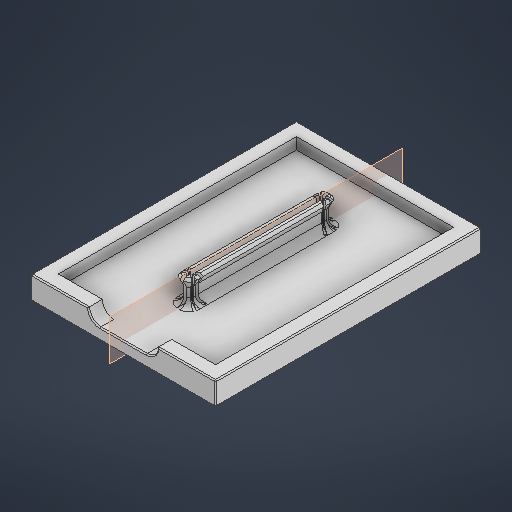
# Autodesk Inventor part: Bolt Slot Covers
Saved by Autodesk Inventor 2026.2 (Build 302298000, 298)
## iProperties
Created: 2026-05-27
Part Number: Bolt Slot Covers
Material: Generic
Document SubType Name: Modeling
Designer: mayhe
Density: 1 g/cm^3
Appearance: Default
Author: mayhe
Autodesk Inventor part; units mm, degrees
ref_plane "XZ Plane" through (0, 0, 0) normal (0, 1, 0) x (-1, 0, 0)
ref_plane "XY Plane" through (0, 0, 0) normal (0, 0, 1) x (1, 0, 0)
sketch "Sketch1" plane through (0, 0, 0) normal (0, 1, 0) x (-1, 0, 0)
  line L0 (40, 57.5) -> (-40, 57.5)
  line L1 (-40, 57.5) -> (-40, -57.5)
  line L2 (-40, -57.5) -> (40, -57.5)
  line L3 (40, -57.5) -> (40, 57.5)
  line L4 (40, 57.5) -> (-40, -57.5) construction
  line L5 (-40, 57.5) -> (40, -57.5) construction
  point P0 (0, 0)
  dimension "d0" = 80
  dimension "d1" = 115
  constraints: 12 end point, 2 midpoint, 2 parallel, 1 horizontal, 1 perpendicular
  measures "d0" distance of L2.end L1.end
  measures "d1" distance of L1.end L0.end
extrude "Extrusion1" add sketch "Sketch1" along normal mid plane 5
sketch "Sketch5" plane through (0, -2.5, 0) normal (0, -1, 0) x (1, 0, 0)
  line L0 (-43.2011, -30.2935) -> (-43.2011, 28.7129) construction
  line L1 (-43.2011, 28.7129) -> (40.8303, 28.7129) construction
  line L2 (40.8303, 28.7129) -> (40.8303, -30.2935) construction
  line L3 (40.8303, -30.2935) -> (-43.2011, -30.2935) construction
  spline S0 degree 2 poles (-3.5733, -17.3493) (-3.5733, -18.0112) (-3.8499, -18.9399) (-4.0475, -19.35) knots 0 0 0 1 2 2 2
  line L4 (-4.0475, -19.35) -> (-5.0652, -19.35)
  line L5 (-5.0652, -19.35) -> (-5.0652, -19.2907)
  spline S1 degree 2 poles (-5.0652, -19.2907) (-4.6897, -18.8905) (-4.2748, -17.8778) (-4.2748, -17.4085) knots 0 0 0 1 2 2 2
  spline S2 degree 2 poles (-4.2748, -17.4085) (-4.2748, -16.7367) (-4.833, -16.05) (-5.2924, -16.05) knots 0 0 0 1 2 2 2
  spline S3 degree 2 poles (-5.2924, -16.05) (-5.658, -16.05) (-6.1125, -16.4106) (-6.2261, -16.8009) knots 0 0 0 1 2 2 2
  spline S4 degree 2 poles (-6.2261, -16.8009) (-6.3051, -17.0825) (-6.4138, -17.5518) (-6.5027, -17.9025) knots 0 0 0 1 2 2 2
  spline S5 degree 2 poles (-6.5027, -17.9025) (-6.5867, -18.2187) (-6.8386, -18.7176) (-7.0412, -18.9103) knots 0 0 0 1 2 2 2
  spline S6 degree 2 poles (-7.0412, -18.9103) (-7.2437, -19.098) (-7.7871, -19.3055) (-8.1428, -19.3055) knots 0 0 0 1 2 2 2
  spline S7 degree 2 poles (-8.1428, -19.3055) (-8.8838, -19.3055) (-9.8866, -18.1495) (-9.8866, -17.2554) knots 0 0 0 1 2 2 2
  spline S8 degree 2 poles (-9.8866, -17.2554) (-9.8866, -16.7416) (-9.6841, -15.8327) (-9.4914, -15.4424) knots 0 0 0 1 2 2 2
  line L6 (-9.4914, -15.4424) -> (-8.5232, -15.4424)
  line L7 (-8.5232, -15.4424) -> (-8.5232, -15.5017)
  spline S9 degree 2 poles (-8.5232, -15.5017) (-8.79, -15.7931) (-9.1852, -16.7021) (-9.1852, -17.2011) knots 0 0 0 1 2 2 2
  spline S10 degree 2 poles (-9.1852, -17.2011) (-9.1852, -17.7642) (-8.6566, -18.4608) (-8.2268, -18.4608) knots 0 0 0 1 2 2 2
  spline S11 degree 2 poles (-8.2268, -18.4608) (-7.8415, -18.4608) (-7.382, -18.0507) (-7.2783, -17.6654) knots 0 0 0 1 2 2 2
  spline S12 degree 2 poles (-7.2783, -17.6654) (-7.2091, -17.4085) (-7.0313, -16.6626) (-6.9572, -16.4156) knots 0 0 0 1 2 2 2
  spline S13 degree 2 poles (-6.9572, -16.4156) (-6.7645, -15.7882) (-5.989, -15.2053) (-5.4209, -15.2053) knots 0 0 0 1 2 2 2
  spline S14 degree 2 poles (-5.4209, -15.2053) (-5.0602, -15.2053) (-4.3686, -15.4967) (-4.1266, -15.7586) knots 0 0 0 1 2 2 2
  spline S15 degree 2 poles (-4.1266, -15.7586) (-3.8598, -16.05) (-3.5733, -16.791) (-3.5733, -17.3493) knots 0 0 0 1 2 2 2
  line L8 (-3.682, -13.6541) -> (-3.682, -14.4248)
  line L9 (-3.682, -14.4248) -> (-10.0497, -14.4248)
  line L10 (-10.0497, -14.4248) -> (-10.0497, -13.6541)
  line L11 (-10.0497, -13.6541) -> (-3.682, -13.6541)
  spline S16 degree 2 poles (-5.9692, -8.7635) (-4.8132, -8.7635) (-3.5535, -9.875) (-3.5535, -10.8037) knots 0 0 0 1 2 2 2
  spline S17 degree 2 poles (-3.5535, -10.8037) (-3.5535, -11.7571) (-4.8527, -12.8489) (-5.9692, -12.8489) knots 0 0 0 1 2 2 2
  spline S18 degree 2 poles (-5.9692, -12.8489) (-7.1153, -12.8489) (-8.3849, -11.7226) (-8.3849, -10.8037) knots 0 0 0 1 2 2 2
  spline S19 degree 2 poles (-8.3849, -10.8037) (-8.3849, -9.875) (-7.1202, -8.7635) (-5.9692, -8.7635) knots 0 0 0 1 2 2 2
  spline S20 degree 2 poles (-5.9692, -9.5588) (-6.8584, -9.5588) (-7.7229, -10.206) (-7.7229, -10.8037) knots 0 0 0 1 2 2 2
  spline S21 degree 2 poles (-7.7229, -10.8037) (-7.7229, -11.4015) (-6.8584, -12.0535) (-5.9692, -12.0535) knots 0 0 0 1 2 2 2
  spline S22 degree 2 poles (-5.9692, -12.0535) (-5.1047, -12.0535) (-4.2155, -11.4015) (-4.2155, -10.8037) knots 0 0 0 1 2 2 2
  spline S23 degree 2 poles (-4.2155, -10.8037) (-4.2155, -10.2109) (-5.0899, -9.5588) (-5.9692, -9.5588) knots 0 0 0 1 2 2 2
  spline S24 degree 2 poles (-3.593, -6.5899) (-3.593, -7.2172) (-4.3093, -7.9237) (-5.0849, -7.9237) knots 0 0 0 1 2 2 2
  line L12 (-5.0849, -7.9237) -> (-7.6192, -7.9237)
  line L13 (-7.6192, -7.9237) -> (-7.6192, -8.4424)
  line L14 (-7.6192, -8.4424) -> (-8.2564, -8.4424)
  line L15 (-8.2564, -8.4424) -> (-8.2564, -7.9237)
  line L16 (-8.2564, -7.9237) -> (-9.5705, -7.9237)
  line L17 (-9.5705, -7.9237) -> (-9.5705, -7.153)
  line L18 (-9.5705, -7.153) -> (-8.2564, -7.153)
  line L19 (-8.2564, -7.153) -> (-8.2564, -5.7352)
  line L20 (-8.2564, -5.7352) -> (-7.6192, -5.7352)
  line L21 (-7.6192, -5.7352) -> (-7.6192, -7.153)
  line L22 (-7.6192, -7.153) -> (-5.4406, -7.153)
  spline S25 degree 2 poles (-5.4406, -7.153) (-5.0948, -7.153) (-4.7144, -7.1283) (-4.5514, -7.0443) knots 0 0 0 1 2 2 2
  spline S26 degree 2 poles (-4.5514, -7.0443) (-4.4081, -6.9752) (-4.2649, -6.664) (-4.2649, -6.3972) knots 0 0 0 1 2 2 2
  spline S27 degree 2 poles (-4.2649, -6.3972) (-4.2649, -6.2095) (-4.3785, -5.8587) (-4.4131, -5.7797) knots 0 0 0 1 2 2 2
  line L23 (-4.4131, -5.7797) -> (-4.4131, -5.7352)
  line L24 (-4.4131, -5.7352) -> (-3.7215, -5.7352)
  spline S28 degree 2 poles (-3.7215, -5.7352) (-3.6622, -5.9526) (-3.593, -6.3972) (-3.593, -6.5899) knots 0 0 0 1 2 2 2
  spline S29 degree 2 poles (-3.5733, -0.1085) (-3.5733, -0.7013) (-3.9734, -1.7042) (-4.3736, -2.0697) knots 0 0 0 1 2 2 2
  spline S30 degree 2 poles (-4.3736, -2.0697) (-4.7688, -2.4353) (-5.9544, -2.8354) (-6.725, -2.8354) knots 0 0 0 1 2 2 2
  spline S31 degree 2 poles (-6.725, -2.8354) (-7.4907, -2.8354) (-8.6269, -2.4452) (-9.0468, -2.0747) knots 0 0 0 1 2 2 2
  spline S32 degree 2 poles (-9.0468, -2.0747) (-9.4569, -1.7091) (-9.8866, -0.7112) (-9.8866, -0.0937) knots 0 0 0 1 2 2 2
  spline S33 degree 2 poles (-9.8866, -0.0937) (-9.8866, 0.2126) (-9.7977, 0.751) (-9.7286, 0.9783) knots 0 0 0 1 2 2 2
  spline S34 degree 2 poles (-9.7286, 0.9783) (-9.6643, 1.1759) (-9.4816, 1.5859) (-9.3729, 1.7884) knots 0 0 0 1 2 2 2
  line L25 (-9.3729, 1.7884) -> (-8.3948, 1.7884)
  line L26 (-8.3948, 1.7884) -> (-8.3948, 1.7242)
  spline S35 degree 2 poles (-8.3948, 1.7242) (-8.4936, 1.6155) (-8.7702, 1.2796) (-8.9036, 1.0375) knots 0 0 0 1 2 2 2
  spline S36 degree 2 poles (-8.9036, 1.0375) (-9.032, 0.8054) (-9.195, 0.257) (-9.195, -0.0987) knots 0 0 0 1 2 2 2
  spline S37 degree 2 poles (-9.195, -0.0987) (-9.195, -0.4889) (-8.8739, -1.1855) (-8.5677, -1.4473) knots 0 0 0 1 2 2 2
  spline S38 degree 2 poles (-8.5677, -1.4473) (-8.2564, -1.7042) (-7.3129, -1.9907) (-6.725, -1.9907) knots 0 0 0 1 2 2 2
  spline S39 degree 2 poles (-6.725, -1.9907) (-6.0976, -1.9907) (-5.1936, -1.6894) (-4.8824, -1.4275) knots 0 0 0 1 2 2 2
  spline S40 degree 2 poles (-4.8824, -1.4275) (-4.581, -1.1706) (-4.2748, -0.484) (-4.2748, -0.0987) knots 0 0 0 1 2 2 2
  spline S41 degree 2 poles (-4.2748, -0.0987) (-4.2748, 0.2521) (-4.4477, 0.8498) (-4.5761, 1.082) knots 0 0 0 1 2 2 2
  spline S42 degree 2 poles (-4.5761, 1.082) (-4.7045, 1.3043) (-4.9713, 1.6353) (-5.0652, 1.7292) knots 0 0 0 1 2 2 2
  line L27 (-5.0652, 1.7292) -> (-5.0652, 1.7884)
  line L28 (-5.0652, 1.7884) -> (-4.0969, 1.7884)
  spline S43 degree 2 poles (-4.0969, 1.7884) (-4.0031, 1.5859) (-3.8302, 1.2302) (-3.7511, 0.9783) knots 0 0 0 1 2 2 2
  spline S44 degree 2 poles (-3.7511, 0.9783) (-3.6622, 0.7115) (-3.5733, 0.257) (-3.5733, -0.1085) knots 0 0 0 1 2 2 2
  spline S45 degree 2 poles (-5.9692, 6.2443) (-4.8132, 6.2443) (-3.5535, 5.1328) (-3.5535, 4.2041) knots 0 0 0 1 2 2 2
  spline S46 degree 2 poles (-3.5535, 4.2041) (-3.5535, 3.2507) (-4.8527, 2.1589) (-5.9692, 2.1589) knots 0 0 0 1 2 2 2
  spline S47 degree 2 poles (-5.9692, 2.1589) (-7.1153, 2.1589) (-8.3849, 3.2853) (-8.3849, 4.2041) knots 0 0 0 1 2 2 2
  spline S48 degree 2 poles (-8.3849, 4.2041) (-8.3849, 5.1328) (-7.1202, 6.2443) (-5.9692, 6.2443) knots 0 0 0 1 2 2 2
  spline S49 degree 2 poles (-5.9692, 5.449) (-6.8584, 5.449) (-7.7229, 4.8019) (-7.7229, 4.2041) knots 0 0 0 1 2 2 2
  spline S50 degree 2 poles (-7.7229, 4.2041) (-7.7229, 3.6064) (-6.8584, 2.9543) (-5.9692, 2.9543) knots 0 0 0 1 2 2 2
  spline S51 degree 2 poles (-5.9692, 2.9543) (-5.1047, 2.9543) (-4.2155, 3.6064) (-4.2155, 4.2041) knots 0 0 0 1 2 2 2
  spline S52 degree 2 poles (-4.2155, 4.2041) (-4.2155, 4.7969) (-5.0899, 5.449) (-5.9692, 5.449) knots 0 0 0 1 2 2 2
  line L29 (-8.2564, 10.6262) -> (-3.682, 8.9021)
  line L30 (-3.682, 8.9021) -> (-3.682, 8.2105)
  line L31 (-3.682, 8.2105) -> (-8.2564, 6.5012)
  line L32 (-8.2564, 6.5012) -> (-8.2564, 7.3361)
  line L33 (-8.2564, 7.3361) -> (-4.7342, 8.5859)
  line L34 (-4.7342, 8.5859) -> (-8.2564, 9.8259)
  line L35 (-8.2564, 9.8259) -> (-8.2564, 10.6262)
  spline S53 degree 2 poles (-3.5782, 13.195) (-3.5782, 12.0983) (-4.8083, 10.8929) (-5.9445, 10.8929) knots 0 0 0 1 2 2 2
  spline S54 degree 2 poles (-5.9445, 10.8929) (-7.0609, 10.8929) (-8.3849, 12.0637) (-8.3849, 13.0072) knots 0 0 0 1 2 2 2
  spline S55 degree 2 poles (-8.3849, 13.0072) (-8.3849, 13.4321) (-8.1379, 14.0891) (-7.876, 14.3312) knots 0 0 0 1 2 2 2
  spline S56 degree 2 poles (-7.876, 14.3312) (-7.6142, 14.5782) (-6.8584, 14.84) (-6.3101, 14.84) knots 0 0 0 1 2 2 2
  line L36 (-6.3101, 14.84) -> (-5.8902, 14.84)
  line L37 (-5.8902, 14.84) -> (-5.8902, 11.6734)
  spline S57 degree 2 poles (-5.8902, 11.6734) (-5.0948, 11.6734) (-4.2501, 12.4737) (-4.2501, 13.1851) knots 0 0 0 1 2 2 2
  spline S58 degree 2 poles (-4.2501, 13.1851) (-4.2501, 13.437) (-4.3637, 13.9261) (-4.4526, 14.1237) knots 0 0 0 1 2 2 2
  spline S59 degree 2 poles (-4.4526, 14.1237) (-4.5514, 14.3312) (-4.7243, 14.6177) (-4.8033, 14.7116) knots 0 0 0 1 2 2 2
  line L38 (-4.8033, 14.7116) -> (-4.8033, 14.756)
  line L39 (-4.8033, 14.756) -> (-3.9635, 14.756)
  spline S60 degree 2 poles (-3.9635, 14.756) (-3.9092, 14.6226) (-3.7511, 14.2176) (-3.7067, 14.0595) knots 0 0 0 1 2 2 2
  spline S61 degree 2 poles (-3.7067, 14.0595) (-3.6424, 13.8372) (-3.5782, 13.4716) (-3.5782, 13.195) knots 0 0 0 1 2 2 2
  spline S62 degree 2 poles (-6.478, 14.0891) (-6.7892, 14.0792) (-7.2437, 13.9508) (-7.3969, 13.8273) knots 0 0 0 1 2 2 2
  spline S63 degree 2 poles (-7.3969, 13.8273) (-7.5698, 13.6939) (-7.7525, 13.274) (-7.7525, 12.9628) knots 0 0 0 1 2 2 2
  spline S64 degree 2 poles (-7.7525, 12.9628) (-7.7525, 12.6565) (-7.5698, 12.2267) (-7.3919, 12.0489) knots 0 0 0 1 2 2 2
  spline S65 degree 2 poles (-7.3919, 12.0489) (-7.2091, 11.876) (-6.7695, 11.6981) (-6.478, 11.6734) knots 0 0 0 1 2 2 2
  line L40 (-6.478, 11.6734) -> (-6.478, 14.0891)
  line L41 (-7.4314, 18.0461) -> (-7.4314, 18.0066)
  spline S66 degree 2 poles (-7.4314, 18.0066) (-7.4561, 17.9176) (-7.466, 17.725) (-7.466, 17.5916) knots 0 0 0 1 2 2 2
  spline S67 degree 2 poles (-7.466, 17.5916) (-7.466, 17.2804) (-7.1943, 16.6678) (-6.9276, 16.3912) knots 0 0 0 1 2 2 2
  line L42 (-6.9276, 16.3912) -> (-3.682, 16.3912)
  line L43 (-3.682, 16.3912) -> (-3.682, 15.6205)
  line L44 (-3.682, 15.6205) -> (-8.2564, 15.6205)
  line L45 (-8.2564, 15.6205) -> (-8.2564, 16.3912)
  line L46 (-8.2564, 16.3912) -> (-7.5747, 16.3912)
  spline S68 degree 2 poles (-7.5747, 16.3912) (-7.9502, 16.8111) (-8.2564, 17.4385) (-8.2564, 17.7349) knots 0 0 0 1 2 2 2
  spline S69 degree 2 poles (-8.2564, 17.7349) (-8.2564, 17.8534) (-8.2466, 17.972) (-8.2317, 18.0461) knots 0 0 0 1 2 2 2
  line L47 (-8.2317, 18.0461) -> (-7.4314, 18.0461)
  spline S70 degree 2 poles (4.3789, -13.4219) (4.8482, -13.4219) (5.6436, -13.7331) (5.9103, -13.995) knots 0 0 0 1 2 2 2
  spline S71 degree 2 poles (5.9103, -13.995) (6.1919, -14.2667) (6.4834, -14.9484) (6.4834, -15.3584) knots 0 0 0 1 2 2 2
  spline S72 degree 2 poles (6.4834, -15.3584) (6.4834, -15.7684) (6.2067, -16.4452) (5.9301, -16.7021) knots 0 0 0 1 2 2 2
  spline S73 degree 2 poles (5.9301, -16.7021) (5.5991, -17.0183) (4.4876, -17.374) (3.6774, -17.374) knots 0 0 0 1 2 2 2
  spline S74 degree 2 poles (3.6774, -17.374) (2.8821, -17.374) (1.6026, -17.0479) (1.1284, -16.707) knots 0 0 0 1 2 2 2
  spline S75 degree 2 poles (1.1284, -16.707) (0.664, -16.3761) (0.1453, -15.3288) (0.1453, -14.6421) knots 0 0 0 1 2 2 2
  spline S76 degree 2 poles (0.1453, -14.6421) (0.1453, -14.4396) (0.1848, -14.0839) (0.2293, -13.9505) knots 0 0 0 1 2 2 2
  line L48 (0.2293, -13.9505) -> (1.0148, -13.9505)
  line L49 (1.0148, -13.9505) -> (1.0148, -13.9851)
  spline S77 degree 2 poles (1.0148, -13.9851) (0.9555, -14.0987) (0.8517, -14.5137) (0.8517, -14.7508) knots 0 0 0 1 2 2 2
  spline S78 degree 2 poles (0.8517, -14.7508) (0.8517, -15.5116) (1.8793, -16.4452) (2.887, -16.5341) knots 0 0 0 1 2 2 2
  spline S79 degree 2 poles (2.887, -16.5341) (2.6845, -16.2427) (2.4622, -15.6301) (2.4622, -15.2646) knots 0 0 0 1 2 2 2
  spline S80 degree 2 poles (2.4622, -15.2646) (2.4622, -14.9089) (2.6055, -14.3754) (2.8228, -14.0839) knots 0 0 0 1 2 2 2
  spline S81 degree 2 poles (2.8228, -14.0839) (3.0748, -13.748) (3.8553, -13.4219) (4.3789, -13.4219) knots 0 0 0 1 2 2 2
  spline S82 degree 2 poles (4.4135, -14.2519) (4.0381, -14.2519) (3.5292, -14.4495) (3.3514, -14.6668) knots 0 0 0 1 2 2 2
  spline S83 degree 2 poles (3.3514, -14.6668) (3.223, -14.8298) (3.139, -15.2349) (3.139, -15.4473) knots 0 0 0 1 2 2 2
  spline S84 degree 2 poles (3.139, -15.4473) (3.139, -15.7339) (3.3119, -16.2723) (3.4749, -16.5341) knots 0 0 0 1 2 2 2
  spline S85 degree 2 poles (3.4749, -16.5341) (3.5638, -16.5391) (3.7318, -16.549) (3.8602, -16.549) knots 0 0 0 1 2 2 2
  spline S86 degree 2 poles (3.8602, -16.549) (4.4925, -16.549) (5.2681, -16.302) (5.4707, -16.1142) knots 0 0 0 1 2 2 2
  spline S87 degree 2 poles (5.4707, -16.1142) (5.6633, -15.9413) (5.8165, -15.5659) (5.8165, -15.3535) knots 0 0 0 1 2 2 2
  spline S88 degree 2 poles (5.8165, -15.3535) (5.8165, -14.8595) (5.115, -14.2519) (4.4135, -14.2519) knots 0 0 0 1 2 2 2
  line L50 (-0.0128, -10.1664) -> (7.6789, -12.5525)
  line L51 (7.6789, -12.5525) -> (7.6789, -13.2441)
  line L52 (7.6789, -13.2441) -> (-0.0128, -10.8679)
  line L53 (-0.0128, -10.8679) -> (-0.0128, -10.1664)
  line L54 (6.3549, -5.7352) -> (6.3549, -9.4946)
  line L55 (6.3549, -9.4946) -> (5.4904, -9.4946)
  spline S89 degree 2 poles (5.4904, -9.4946) (5.1101, -9.0895) (4.4036, -8.3683) (4.0232, -8.0225) knots 0 0 0 1 2 2 2
  spline S90 degree 2 poles (4.0232, -8.0225) (3.2575, -7.3259) (2.3387, -6.8171) (1.8496, -6.8171) knots 0 0 0 1 2 2 2
  spline S91 degree 2 poles (1.8496, -6.8171) (1.5928, -6.8171) (1.2074, -6.9752) (1.0839, -7.1184) knots 0 0 0 1 2 2 2
  spline S92 degree 2 poles (1.0839, -7.1184) (0.9604, -7.2617) (0.8369, -7.6371) (0.8369, -7.8644) knots 0 0 0 1 2 2 2
  spline S93 degree 2 poles (0.8369, -7.8644) (0.8369, -8.0818) (0.9456, -8.5264) (1.0296, -8.7289) knots 0 0 0 1 2 2 2
  spline S94 degree 2 poles (1.0296, -8.7289) (1.0987, -8.9018) (1.2963, -9.2229) (1.3655, -9.3217) knots 0 0 0 1 2 2 2
  line L56 (1.3655, -9.3217) -> (1.3655, -9.3662)
  line L57 (1.3655, -9.3662) -> (0.4961, -9.3662)
  spline S95 degree 2 poles (0.4961, -9.3662) (0.3726, -9.1142) (0.1305, -8.2102) (0.1305, -7.8051) knots 0 0 0 1 2 2 2
  spline S96 degree 2 poles (0.1305, -7.8051) (0.1305, -6.9505) (1.0345, -5.9872) (1.8052, -5.9872) knots 0 0 0 1 2 2 2
  spline S97 degree 2 poles (1.8052, -5.9872) (2.1658, -5.9872) (2.7685, -6.1551) (3.0254, -6.3033) knots 0 0 0 1 2 2 2
  spline S98 degree 2 poles (3.0254, -6.3033) (3.2921, -6.4515) (3.8158, -6.8813) (4.0677, -7.1184) knots 0 0 0 1 2 2 2
  spline S99 degree 2 poles (4.0677, -7.1184) (4.4876, -7.5038) (5.3867, -8.4473) (5.6485, -8.7289) knots 0 0 0 1 2 2 2
  line L58 (5.6485, -8.7289) -> (5.6485, -5.7352)
  line L59 (5.6485, -5.7352) -> (6.3549, -5.7352)
  line L60 (-0.0128, -2.3859) -> (7.6789, -4.7719)
  line L61 (7.6789, -4.7719) -> (7.6789, -5.4635)
  line L62 (7.6789, -5.4635) -> (-0.0128, -3.0874)
  line L63 (-0.0128, -3.0874) -> (-0.0128, -2.3859)
  line L64 (6.3549, 2.0453) -> (6.3549, -1.7141)
  line L65 (6.3549, -1.7141) -> (5.4904, -1.7141)
  spline S100 degree 2 poles (5.4904, -1.7141) (5.1101, -1.309) (4.4036, -0.5877) (4.0232, -0.2419) knots 0 0 0 1 2 2 2
  spline S101 degree 2 poles (4.0232, -0.2419) (3.2575, 0.4546) (2.3387, 0.9634) (1.8496, 0.9634) knots 0 0 0 1 2 2 2
  spline S102 degree 2 poles (1.8496, 0.9634) (1.5928, 0.9634) (1.2074, 0.8054) (1.0839, 0.6621) knots 0 0 0 1 2 2 2
  spline S103 degree 2 poles (1.0839, 0.6621) (0.9604, 0.5188) (0.8369, 0.1434) (0.8369, -0.0838) knots 0 0 0 1 2 2 2
  spline S104 degree 2 poles (0.8369, -0.0838) (0.8369, -0.3012) (0.9456, -0.7458) (1.0296, -0.9483) knots 0 0 0 1 2 2 2
  spline S105 degree 2 poles (1.0296, -0.9483) (1.0987, -1.1212) (1.2963, -1.4423) (1.3655, -1.5411) knots 0 0 0 1 2 2 2
  line L66 (1.3655, -1.5411) -> (1.3655, -1.5856)
  line L67 (1.3655, -1.5856) -> (0.4961, -1.5856)
  spline S106 degree 2 poles (0.4961, -1.5856) (0.3726, -1.3337) (0.1305, -0.4296) (0.1305, -0.0246) knots 0 0 0 1 2 2 2
  spline S107 degree 2 poles (0.1305, -0.0246) (0.1305, 0.8301) (1.0345, 1.7934) (1.8052, 1.7934) knots 0 0 0 1 2 2 2
  spline S108 degree 2 poles (1.8052, 1.7934) (2.1658, 1.7934) (2.7685, 1.6254) (3.0254, 1.4772) knots 0 0 0 1 2 2 2
  spline S109 degree 2 poles (3.0254, 1.4772) (3.2921, 1.329) (3.8158, 0.8992) (4.0677, 0.6621) knots 0 0 0 1 2 2 2
  spline S110 degree 2 poles (4.0677, 0.6621) (4.4876, 0.2768) (5.3867, -0.6668) (5.6485, -0.9483) knots 0 0 0 1 2 2 2
  line L68 (5.6485, -0.9483) -> (5.6485, 2.0453)
  line L69 (5.6485, 2.0453) -> (6.3549, 2.0453)
  spline S111 degree 2 poles (3.3069, 6.6544) (4.947, 6.6544) (6.4834, 5.7009) (6.4834, 4.708) knots 0 0 0 1 2 2 2
  spline S112 degree 2 poles (6.4834, 4.708) (6.4834, 3.7002) (4.9174, 2.7567) (3.3119, 2.7567) knots 0 0 0 1 2 2 2
  spline S113 degree 2 poles (3.3119, 2.7567) (1.6619, 2.7567) (0.1354, 3.7101) (0.1354, 4.708) knots 0 0 0 1 2 2 2
  spline S114 degree 2 poles (0.1354, 4.708) (0.1354, 5.7108) (1.7163, 6.6544) (3.3069, 6.6544) knots 0 0 0 1 2 2 2
  spline S115 degree 2 poles (5.1644, 5.6071) (4.8631, 5.7256) (3.9343, 5.8244) (3.3069, 5.8244) knots 0 0 0 1 2 2 2
  spline S116 degree 2 poles (3.3069, 5.8244) (2.6796, 5.8244) (1.7558, 5.7256) (1.4445, 5.6021) knots 0 0 0 1 2 2 2
  spline S117 degree 2 poles (1.4445, 5.6021) (1.1333, 5.4786) (0.8122, 5.0489) (0.8122, 4.708) knots 0 0 0 1 2 2 2
  spline S118 degree 2 poles (0.8122, 4.708) (0.8122, 4.3671) (1.1333, 3.9275) (1.4544, 3.799) knots 0 0 0 1 2 2 2
  spline S119 degree 2 poles (1.4544, 3.799) (1.7657, 3.6755) (2.7141, 3.5866) (3.3119, 3.5866) knots 0 0 0 1 2 2 2
  spline S120 degree 2 poles (3.3119, 3.5866) (3.9541, 3.5866) (4.8137, 3.6656) (5.1496, 3.7941) knots 0 0 0 1 2 2 2
  spline S121 degree 2 poles (5.1496, 3.7941) (5.4657, 3.9126) (5.8066, 4.3523) (5.8066, 4.708) knots 0 0 0 1 2 2 2
  spline S122 degree 2 poles (5.8066, 4.708) (5.8066, 5.0439) (5.4855, 5.4836) (5.1644, 5.6071) knots 0 0 0 1 2 2 2
  line L70 (6.3549, 11.1943) -> (6.3549, 7.4349)
  line L71 (6.3549, 7.4349) -> (5.4904, 7.4349)
  spline S123 degree 2 poles (5.4904, 7.4349) (5.1101, 7.84) (4.4036, 8.5612) (4.0232, 8.907) knots 0 0 0 1 2 2 2
  spline S124 degree 2 poles (4.0232, 8.907) (3.2575, 9.6036) (2.3387, 10.1124) (1.8496, 10.1124) knots 0 0 0 1 2 2 2
  spline S125 degree 2 poles (1.8496, 10.1124) (1.5928, 10.1124) (1.2074, 9.9543) (1.0839, 9.811) knots 0 0 0 1 2 2 2
  spline S126 degree 2 poles (1.0839, 9.811) (0.9604, 9.6678) (0.8369, 9.2923) (0.8369, 9.0651) knots 0 0 0 1 2 2 2
  spline S127 degree 2 poles (0.8369, 9.0651) (0.8369, 8.8477) (0.9456, 8.4031) (1.0296, 8.2006) knots 0 0 0 1 2 2 2
  spline S128 degree 2 poles (1.0296, 8.2006) (1.0987, 8.0277) (1.2963, 7.7066) (1.3655, 7.6078) knots 0 0 0 1 2 2 2
  line L72 (1.3655, 7.6078) -> (1.3655, 7.5633)
  line L73 (1.3655, 7.5633) -> (0.4961, 7.5633)
  spline S129 degree 2 poles (0.4961, 7.5633) (0.3726, 7.8153) (0.1305, 8.7193) (0.1305, 9.1244) knots 0 0 0 1 2 2 2
  spline S130 degree 2 poles (0.1305, 9.1244) (0.1305, 9.979) (1.0345, 10.9423) (1.8052, 10.9423) knots 0 0 0 1 2 2 2
  spline S131 degree 2 poles (1.8052, 10.9423) (2.1658, 10.9423) (2.7685, 10.7744) (3.0254, 10.6262) knots 0 0 0 1 2 2 2
  spline S132 degree 2 poles (3.0254, 10.6262) (3.2921, 10.478) (3.8158, 10.0482) (4.0677, 9.811) knots 0 0 0 1 2 2 2
  spline S133 degree 2 poles (4.0677, 9.811) (4.4876, 9.4257) (5.3867, 8.4822) (5.6485, 8.2006) knots 0 0 0 1 2 2 2
  line L74 (5.6485, 8.2006) -> (5.6485, 11.1943)
  line L75 (5.6485, 11.1943) -> (6.3549, 11.1943)
  spline S134 degree 2 poles (4.3789, 15.8626) (4.8482, 15.8626) (5.6436, 15.5514) (5.9103, 15.2895) knots 0 0 0 1 2 2 2
  spline S135 degree 2 poles (5.9103, 15.2895) (6.1919, 15.0178) (6.4834, 14.3361) (6.4834, 13.9261) knots 0 0 0 1 2 2 2
  spline S136 degree 2 poles (6.4834, 13.9261) (6.4834, 13.5161) (6.2067, 12.8393) (5.9301, 12.5824) knots 0 0 0 1 2 2 2
  spline S137 degree 2 poles (5.9301, 12.5824) (5.5991, 12.2662) (4.4876, 11.9106) (3.6774, 11.9106) knots 0 0 0 1 2 2 2
  spline S138 degree 2 poles (3.6774, 11.9106) (2.8821, 11.9106) (1.6026, 12.2366) (1.1284, 12.5775) knots 0 0 0 1 2 2 2
  spline S139 degree 2 poles (1.1284, 12.5775) (0.664, 12.9084) (0.1453, 13.9557) (0.1453, 14.6424) knots 0 0 0 1 2 2 2
  spline S140 degree 2 poles (0.1453, 14.6424) (0.1453, 14.8449) (0.1848, 15.2006) (0.2293, 15.334) knots 0 0 0 1 2 2 2
  line L76 (0.2293, 15.334) -> (1.0148, 15.334)
  line L77 (1.0148, 15.334) -> (1.0148, 15.2994)
  spline S141 degree 2 poles (1.0148, 15.2994) (0.9555, 15.1858) (0.8517, 14.7708) (0.8517, 14.5337) knots 0 0 0 1 2 2 2
  spline S142 degree 2 poles (0.8517, 14.5337) (0.8517, 13.773) (1.8793, 12.8393) (2.887, 12.7504) knots 0 0 0 1 2 2 2
  spline S143 degree 2 poles (2.887, 12.7504) (2.6845, 13.0418) (2.4622, 13.6544) (2.4622, 14.02) knots 0 0 0 1 2 2 2
  spline S144 degree 2 poles (2.4622, 14.02) (2.4622, 14.3756) (2.6055, 14.9092) (2.8228, 15.2006) knots 0 0 0 1 2 2 2
  spline S145 degree 2 poles (2.8228, 15.2006) (3.0748, 15.5365) (3.8553, 15.8626) (4.3789, 15.8626) knots 0 0 0 1 2 2 2
  spline S146 degree 2 poles (4.4135, 15.0327) (4.0381, 15.0327) (3.5292, 14.8351) (3.3514, 14.6177) knots 0 0 0 1 2 2 2
  spline S147 degree 2 poles (3.3514, 14.6177) (3.223, 14.4547) (3.139, 14.0496) (3.139, 13.8372) knots 0 0 0 1 2 2 2
  spline S148 degree 2 poles (3.139, 13.8372) (3.139, 13.5507) (3.3119, 13.0122) (3.4749, 12.7504) knots 0 0 0 1 2 2 2
  spline S149 degree 2 poles (3.4749, 12.7504) (3.5638, 12.7454) (3.7318, 12.7355) (3.8602, 12.7355) knots 0 0 0 1 2 2 2
  spline S150 degree 2 poles (3.8602, 12.7355) (4.4925, 12.7355) (5.2681, 12.9825) (5.4707, 13.1703) knots 0 0 0 1 2 2 2
  spline S151 degree 2 poles (5.4707, 13.1703) (5.6633, 13.3432) (5.8165, 13.7186) (5.8165, 13.931) knots 0 0 0 1 2 2 2
  spline S152 degree 2 poles (5.8165, 13.931) (5.8165, 14.425) (5.115, 15.0327) (4.4135, 15.0327) knots 0 0 0 1 2 2 2
  point P0 (0, 0)
  dimension "d0" = 80
  dimension "d1" = 115
  constraints: 2 other
extrude "Text" cut sketch "Sketch5" against normal blind 1
sketch "Sketch6" plane through (0, 2.5, 0) normal (0, 1, 0) x (1, 0, 0)
  line L0 (-40, -57.5) -> (40, -57.5) projected
  line L1 (-40, 57.5) -> (-40, -57.5) projected
  line L2 (-40, -57.5) -> (40, -57.5) projected
  line L3 (40, -57.5) -> (40, 57.5) projected
  line L4 (40, 57.5) -> (-40, 57.5) projected
  line L5 (-34, -51.5) -> (-34, 51.5)
  line L6 (-34, 51.5) -> (34, 51.5)
  line L7 (34, 51.5) -> (34, -51.5)
  line L8 (34, -51.5) -> (-34, -51.5)
  line L9 (0, -51.5) -> (0, -57.5)
  line L10 (-15, -51.5) -> (15, -51.5)
  line L11 (15, -51.5) -> (15, -57.5)
  line L12 (15, -57.5) -> (-15, -57.5)
  line L13 (-15, -57.5) -> (-15, -51.5)
  line L14 (-15, -51.5) -> (15, -57.5) construction
  line L15 (15, -51.5) -> (-15, -57.5) construction
  point P0 (0, 0)
  point P1 (0, -54.5)
  point P2 (-15, -51.5)
  point P3 (15, -51.5)
  dimension "d31" = 6
  dimension "d32" = 30
  constraints: 22 end point, 5 midpoint, 2 parallel, 1 horizontal, 1 perpendicular, 1 point on line, 3 other
  measures "d31" distance between parallel lines of L1 L5
  measures "d32" distance of L11.end L12.end
extrude "Extrusion6" add sketch "Sketch6" along normal blind 5 contours L1 L4 L3 L0 L11 L8 L7 L6 L5 L13
sketch "Sketch7" plane through (0, 2.5, 0) normal (0, 1, 0) x (1, 0, 0)
  line L0 (0, 29) -> (0, -29) construction
  line L1 (-1.75, 29) -> (-1.75, -29)
  line L2 (1.75, -29) -> (1.75, 29)
  arc A0 (1.75, 29) -> (-1.75, 29) centre (0, 29) ccw
  arc A1 (-1.75, -29) -> (1.75, -29) centre (0, -29) ccw
  point P0 (0, 0)
  dimension "d35" = 29
  dimension "d36" = 3.5
  constraints: 8 end point, 4 point on circle, 4 tangent, 2 centre point, 1 midpoint, 1 parallel, 1 vertical
  measures "d35" distance of point (0, 0) L0.end
  measures "d36" diameter of A1
extrude "Extrusion7" add sketch "Sketch7" along normal blind 7
sketch "Sketch8" plane through (0, 9.5, 0) normal (0, 1, 0) x (1, 0, 0)
  arc A0 (-1.75, -29) -> (1.75, -29) centre (0, -29) ccw projected
  line L0 (1.75, -29) -> (1.75, 29) projected
  arc A1 (1.75, 29) -> (-1.75, 29) centre (0, 29) ccw projected
  line L1 (-1.75, 29) -> (-1.75, -29) projected
  arc A2 (-3.25, -29) -> (3.25, -29) centre (0, -29) ccw
  line L2 (-3.25, -29) -> (-3.25, 29)
  arc A3 (3.25, 29) -> (-3.25, 29) centre (0, 29) ccw
  line L3 (3.25, 29) -> (3.25, -29)
  point P0 (0, 0)
  dimension "d40" = 1.5
  constraints: 4 end point, 4 point on circle, 2 centre point, 3 other
  measures "d40" radial gap between concentric circles of A0 A2
extrude "Knob Width" add sketch "Sketch8" along normal blind 4 contours L1 A1 L0 A0 | L2 A3 L3 A2
chamfer "Chamfer3" distance 1.5 distance2 3 4 edges at (-3.25, 9.5, 0) (0, 9.5, 32.25) (3.25, 9.5, 0) (0, 9.5, -32.25) measured on face at (2.75, 9.5, 0) measured on face at (0, 9.5, -31.75) measured on face at (0, 9.5, 31.75) measured on face at (-2.75, 9.5, 0)
chamfer "Chamfer4" distance 1 distance2 1 4 edges at (-3.25, 13.5, 0) (0, 13.5, 32.25) (3.25, 13.5, 0) (0, 13.5, -32.25) measured on face at (-2.75, 13.5, 0) measured on face at (2.75, 13.5, 0) measured on face at (0, 13.5, -31.75) measured on face at (0, 13.5, 31.75)
fillet "Fillet3" radius 3 4 edges at (0, 2.5, -30.75) (1.75, 2.5, 0) (0, 2.5, 30.75) (-1.75, 2.5, 0)
sketch "Sketch9" plane through (0, 13.5, 0) normal (0, 1, 0) x (1, 0, 0)
  line L0 (-0.625, 37.5) -> (0.625, 37.5)
  line L1 (0.625, 37.5) -> (0.625, -37.5)
  line L2 (0.625, -37.5) -> (-0.625, -37.5)
  line L3 (-0.625, 37.5) -> (0.625, -37.5) construction
  line L4 (0.625, 37.5) -> (-0.625, -37.5) construction
  line L5 (-3.9551, -25.4912) -> (4.7051, -30.4912)
  line L6 (4.7051, -30.4912) -> (4.2051, -31.3572)
  line L7 (4.2051, -31.3572) -> (-4.4551, -26.3572)
  line L8 (-4.4551, -26.3572) -> (-3.9551, -25.4912)
  line L9 (-3.9551, -25.4912) -> (4.2051, -31.3572) construction
  line L10 (4.7051, -30.4912) -> (-4.4551, -26.3572) construction
  line L11 (-3.9551, -25.4912) -> (6.0449, -25.4912) construction
  arc A0 (-3.25, -29) -> (3.25, -29) centre (0, -29) ccw projected
  line L12 (0, -32.25) -> (0, 0)
  line L13 (-1.75, 29) -> (-1.75, -29) projected
  line L14 (-4.75, 29) -> (-4.75, -29) projected
  line L15 (-4.75, 0) -> (4.25, 0)
  line L16 (3.9551, -25.4912) -> (-4.7051, -30.4912)
  line L17 (-4.7051, -30.4912) -> (-4.2051, -31.3572)
  line L18 (-4.2051, -31.3572) -> (4.4551, -26.3572)
  line L19 (4.4551, -26.3572) -> (3.9551, -25.4912)
  line L20 (-0.625, -37.5) -> (-0.625, 37.5)
  line L21 (-3.9551, 25.4912) -> (4.7051, 30.4912)
  line L22 (4.7051, 30.4912) -> (4.2051, 31.3572)
  line L23 (4.2051, 31.3572) -> (-4.4551, 26.3572)
  line L24 (-4.4551, 26.3572) -> (-3.9551, 25.4912)
  line L25 (3.9551, 25.4912) -> (-4.7051, 30.4912)
  line L26 (4.4551, 26.3572) -> (3.9551, 25.4912)
  line L27 (-4.2051, 31.3572) -> (4.4551, 26.3572)
  line L28 (-4.7051, 30.4912) -> (-4.2051, 31.3572)
  point P0 (0.125, -28.4242)
  point P1 (-0.625, -27.4138)
  point P2 (-1, -28.352)
  point P3 (-0.625, -29.2902)
  point P4 (0.625, -29.2902)
  point P5 (1, -28.352)
  point P6 (0.625, -27.4138)
  point P7 (0.625, 27.4138)
  point P8 (1, 28.352)
  point P9 (0.625, 29.2902)
  point P10 (-0.625, 29.2902)
  point P11 (-1, 28.352)
  point P12 (-0.625, 27.4138)
  dimension "d50" = 1.25
  dimension "d52" = 10
  dimension "d53" = 30
  dimension "d54" = 1
  dimension "d55" = 75
  constraints: 54 end point, 12 symmetric about line, 5 midpoint, 5 parallel, 2 horizontal, 2 perpendicular, 1 equal length, 1 point on circle
  measures "d50" distance of L1.end L2.end
  measures "d52" distance of L5.start L5.end
  measures "d53" angle of L5 L11
  measures "d54" distance of L5.end L6.end
  measures "d55" distance between parallel lines of L2 L0
extrude "Extrusion9" cut sketch "Sketch9" against normal up to surface (11 mm away) contours L0 L1 L23 L27 L20 | L27 L23 L20 | L20 L23 L25 L28 L27 | L23 L22 L21 L27 L1 | L1 L27 L23 | L23 L27 L1 L21 L25 L20 | L20 L25 L23 | L27 L21 L1 | L25 L21 L20 | L20 L21 L13 L23 L25 | L21 L27 L26 L25 L1 | L1 L25 L21 | L21 L25 L1 L15 L20 | L13 L21 L24 L23 | L15 L12 L5 L20 | L1 L16 L12 L15 | L20 L16 L7 L13 L5 | L5 L16 L20 | L16 L19 L18 L5 L1 | L1 L5 L16 | L13 L7 L8 L5 | L5 L1 L18 L12 | L12 L7 L20 L16 | L20 L7 L16 | L5 L18 L1 | L18 L1 L7 | L18 L20 L7 | L7 L1 A0 L12 | L12 A0 L20 L18 | L7 L20 L18 A0 L16 | L18 L5 A0 L7 L1 | A0 L1 L2 L20 | L5 L6 L7 A0 | A0 L18 L17 L16
draft "FaceDraft2" angle -2.5 pull direction (0, -1, 0) faces at (-0.625, 9.8333, -9.1379) fixed edges at (-0.625, 2.5, 0)
draft "FaceDraft3" angle -2.5 pull direction (0, -1, 0) faces at (0.625, 9.8333, 9.1379) fixed edges at (0.625, 2.5, 0)
fillet "Fillet4" radius 0.5 2 edges at (-0.625, 2.5, 0) (0.625, 2.5, 0)
fillet "Fillet5" radius 5 2 edges at (-15, 2.5, 54.5) (15, 2.5, 54.5)
chamfer "Chamfer2" distance 0.5 angle 45 18 edges at (0, -2.5, 57.5) (40, -2.5, 0) (-40, -2.5, 0) (0, -2.5, -57.5) (-40, 2.5, 57.5) (40, 2.5, 57.5) (40, 2.5, -57.5) (-40, 2.5, -57.5) (-40, 7.5, 0) (0, 7.5, -57.5) (40, 7.5, 0) (15, 7.5, 57.5) (27.5, 7.5, 57.5) (-15, 7.5, 57.5) (-27.5, 7.5, 57.5) (-13.5356, 3.9644, 57.5) (0, 2.5, 57.5) (13.5356, 3.9644, 57.5)
body "Solid1"
